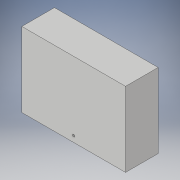
# Autodesk Inventor part: Regulator2
Saved by Autodesk Inventor 2017 (Build 210142000, 142)
## iProperties
Created: 2018-07-29
Part Number: Regulator2
Material: Generic
Document SubType Name: Modeling
Designer: Alexander Miller
Density: 1 g/cm^3
Appearance: Default
Author: Alexander Miller
Autodesk Inventor part; units mm, degrees
ref_plane "YZ Plane" through (0, 0, 0) normal (1, 0, 0) x (0, 1, 0)
ref_plane "XZ Plane" through (0, 0, 0) normal (0, 1, 0) x (-1, 0, 0)
ref_plane "XY Plane" through (0, 0, 0) normal (0, 0, 1) x (1, 0, 0)
sketch "Sketch1" plane through (0, 0, 0) normal (0, 0, 1) x (1, 0, 0)
  line L0 (-22.25, 16) -> (22.25, 16)
  line L1 (22.25, 16) -> (22.25, -16)
  line L2 (22.25, -16) -> (-22.25, -16)
  line L3 (-22.25, -16) -> (-22.25, 16)
  circle A0 centre (0, -13.46) radius 0.5
  point P0 (0, 0)
  point P1 (0, 16)
  point P2 (22.25, 0)
  dimension "d0" = 44.5
  dimension "d1" = 32
  dimension "d4" = 1
  dimension "d5" = 2.54
  constraints: 8 end point, 2 midpoint, 2 parallel, 2 vertical alignment, 1 centre point, 1 horizontal, 1 horizontal alignment, 1 perpendicular
  measures "d0" distance of L0.start L0.end
  measures "d1" distance of L0.end L1.end
  measures "d4" diameter of A0
  measures "d5" distance from line of A0.centre L2
extrude "Extrusion1" add sketch "Sketch1" along normal blind 14
body "Solid1"
